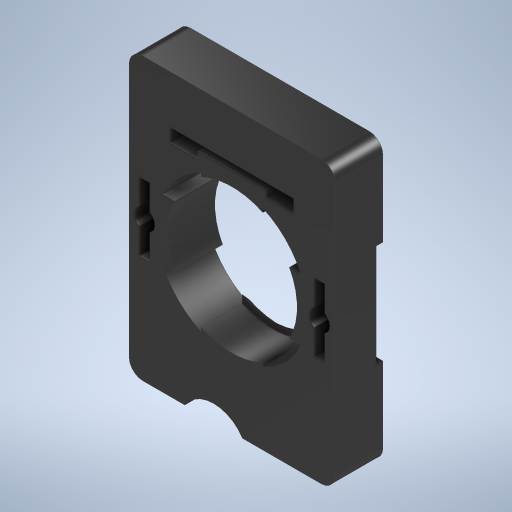
# Autodesk Inventor part: BASE
Saved by Autodesk Inventor 2023 (Build 270158000, 158)
## iProperties
Created: 2023-10-18
Part Number: BASE
Material: Genérico
Document SubType Name: Modeling
Designer: vinicius.sena
Density: 1 g/cm^3
Appearance: Padrão
Author: vinicius.sena
Autodesk Inventor part; units mm, degrees
ref_plane "YZ Plane" through (0, 0, 0) normal (1, 0, 0) x (0, 1, 0)
ref_plane "XZ Plane" through (0, 0, 0) normal (0, 1, 0) x (-1, 0, 0)
ref_plane "XY Plane" through (0, 0, 0) normal (0, 0, 1) x (1, 0, 0)
sketch "Esboço1" plane through (0, 0, 0) normal (0, 0, 1) x (1, 0, 0)
  line L0 (-15, 20.5) -> (15, 20.5)
  line L1 (15, 20.5) -> (15, -20.5)
  line L2 (15, -20.5) -> (-15, -20.5)
  line L3 (-15, -20.5) -> (-15, 20.5)
  line L4 (-15, 20.5) -> (15, -20.5) construction
  line L5 (15, 20.5) -> (-15, -20.5) construction
  point P0 (0, 0)
  dimension "d0" = 30
  dimension "d1" = 41
  constraints: 12 end point, 2 midpoint, 2 parallel, 1 horizontal, 1 perpendicular
  measures "d0" distance of L1.end L2.end
  measures "d1" distance of L0.end L1.end
extrude "Extrusão1" add sketch "Esboço1" along normal blind 7
sketch "Esboço2" plane through (0, 0, 7) normal (0, 0, 1) x (1, 0, 0)
  circle A0 centre (0, 0) radius 11
  dimension "d4" = 22
  constraints: 1 centre point, 1 coincident
  measures "d4" diameter of A0
extrude "Extrusão2" cut sketch "Esboço2" against normal blind 7
sketch "Esboço3" plane through (0, 0, 7) normal (0, 0, 1) x (1, 0, 0)
  circle A0 centre (-2.6743, -23.2026) radius 5
  point P0 (0, 0)
  dimension "d7" = 10
  constraints: 1 centre point
  measures "d7" diameter of A0
extrude "Extrusão3" cut sketch "Esboço3" against normal through all
sketch "Esboço5" plane through (0, 0, 7) normal (0, 0, 1) x (1, 0, 0)
  line L0 (-13.5, 5) -> (-12, 5)
  line L1 (-12, 5) -> (-12, -5)
  line L2 (-12, -5) -> (-13.5, -5)
  line L3 (-13.5, -5) -> (-13.5, 5)
  line L4 (-13.5, 5) -> (-12, -5) construction
  line L5 (-12, 5) -> (-13.5, -5) construction
  line L6 (12, 5) -> (13.5, 5)
  line L7 (13.5, 5) -> (13.5, -5)
  line L8 (13.5, -5) -> (12, -5)
  line L9 (12, -5) -> (12, 5)
  line L10 (12, 5) -> (13.5, -5) construction
  line L11 (13.5, 5) -> (12, -5) construction
  line L12 (15, -20.5) -> (15, 20.5) projected
  line L13 (-15, 20.5) -> (-15, -20.5) projected
  point P0 (0, 0)
  point P1 (-12.75, 0)
  point P2 (12.75, 0)
  dimension "d10" = 1.5
  dimension "d11" = 10
  dimension "d12" = 1.5
  dimension "d13" = 10
  dimension "d14" = 1.5
  dimension "d15" = 1.5
  constraints: 24 end point, 4 midpoint, 4 parallel, 2 horizontal, 2 perpendicular
  measures "d10" distance of L1.end L2.end
  measures "d11" distance of L0.end L1.end
  measures "d12" distance of L7.end L8.end
  measures "d13" distance of L6.end L7.end
  measures "d14" distance between parallel lines of L12 L7
  measures "d15" distance between parallel lines of L13 L3
extrude "Extrusão4" cut sketch "Esboço5" against normal through all
sketch "Esboço6" plane through (0, 0, 7) normal (0, 0, 1) x (1, 0, 0)
  circle A0 centre (12.75, 0) radius 1.5
  circle A1 centre (-12.75, 0) radius 1.5
  line L0 (-13.5, 5) -> (-12, 5) projected
  line L1 (12, 5) -> (13.5, 5) projected
  point P0 (0, 0)
  point P1 (-12.75, 5)
  point P2 (12.75, 5)
  dimension "d18" = 3
  dimension "d19" = 3
  dimension "d20" = 0
  dimension "d21" = 0
  constraints: 2 centre point, 2 midpoint
  measures "d18" diameter of A0
  measures "d19" diameter of A1
  measures "d20" horizontal distance of point (-12.75, 5) A1.centre
  measures "d21" horizontal distance of point (12.75, 5) A0.centre
extrude "Extrusão5" cut sketch "Esboço6" against normal through all
sketch "Esboço7" plane through (0, 0, 7) normal (0, 0, 1) x (1, 0, 0)
  circle A0 centre (0, 0) radius 9.5
  circle A1 centre (0, 0) radius 11
  line L0 (-15, 4.5) -> (15, 4.5)
  line L1 (15, 4.5) -> (15, -4.5)
  line L2 (15, -4.5) -> (-15, -4.5)
  line L3 (-15, -4.5) -> (-15, 4.5)
  line L4 (-15, 4.5) -> (15, -4.5) construction
  line L5 (15, 4.5) -> (-15, -4.5) construction
  line L6 (-4.5, -15) -> (4.5, -15)
  line L7 (4.5, -15) -> (4.5, 15)
  line L8 (4.5, 15) -> (-4.5, 15)
  line L9 (-4.5, 15) -> (-4.5, -15)
  line L10 (-4.5, -15) -> (4.5, 15) construction
  line L11 (4.5, -15) -> (-4.5, 15) construction
  point P0 (8.3666, -4.5)
  point P1 (10.0374, -4.5)
  point P2 (10.0374, 4.5)
  point P3 (8.3666, 4.5)
  point P4 (-4.5, -8.3666)
  point P5 (-4.5, -10.0374)
  point P6 (4.5, -10.0374)
  point P7 (4.5, -8.3666)
  point P8 (-10.0374, -4.5)
  point P9 (-8.3666, -4.5)
  point P10 (-8.3666, 4.5)
  point P11 (-10.0374, 4.5)
  point P12 (-4.5, 10.0374)
  point P13 (-4.5, 8.3666)
  point P14 (4.5, 8.3666)
  point P15 (4.5, 10.0374)
  dimension "d24" = 19
  dimension "d25" = 22
  dimension "d26" = 30
  dimension "d27" = 9
  dimension "d28" = 9
  dimension "d29" = 30
  constraints: 24 end point, 4 midpoint, 4 parallel, 2 centre point, 2 coincident, 2 horizontal, 2 perpendicular
  measures "d24" diameter of A0
  measures "d25" diameter of A1
  measures "d26" distance of L1.end L2.end
  measures "d27" distance of L0.end L1.end
  measures "d28" distance of L8.end L7.end
  measures "d29" distance of L7.end L6.end
extrude "Extrusão6" add sketch "Esboço7" against normal blind 7 contours A0 L0 A1 L2 | A0 L9 A1 L7 | L7 A1 L9 A0 | A0 L2 A1 L0
sketch "Esboço8" plane through (0, 0, 7) normal (0, 0, 1) x (1, 0, 0)
  circle A0 centre (0, 0) radius 11
  circle A1 centre (0, 0) radius 10.5
  circle A2 centre (0, 0) radius 9.5
  line L0 (-4.5, 15) -> (4.5, 15)
  line L1 (4.5, 15) -> (4.5, -15)
  line L2 (4.5, -15) -> (-4.5, -15)
  line L3 (-4.5, -15) -> (-4.5, 15)
  line L4 (-4.5, 15) -> (4.5, -15) construction
  line L5 (4.5, 15) -> (-4.5, -15) construction
  line L6 (-15, 4.5) -> (15, 4.5)
  line L7 (15, 4.5) -> (15, -4.5)
  line L8 (15, -4.5) -> (-15, -4.5)
  line L9 (-15, -4.5) -> (-15, 4.5)
  line L10 (-15, 4.5) -> (15, -4.5) construction
  line L11 (15, 4.5) -> (-15, -4.5) construction
  point P0 (-4.5, -8.3666)
  point P1 (-4.5, -9.4868)
  point P2 (4.5, -9.4868)
  point P3 (4.5, -8.3666)
  point P4 (8.3666, -4.5)
  point P5 (9.4868, -4.5)
  point P6 (9.4868, 4.5)
  point P7 (8.3666, 4.5)
  point P8 (-9.4868, -4.5)
  point P9 (-8.3666, -4.5)
  point P10 (-8.3666, 4.5)
  point P11 (-9.4868, 4.5)
  point P12 (-4.5, 9.4868)
  point P13 (-4.5, 8.3666)
  point P14 (4.5, 8.3666)
  point P15 (4.5, 9.4868)
  dimension "d32" = 22
  dimension "d33" = 21
  dimension "d34" = 19
  dimension "d35" = 9
  dimension "d36" = 30
  dimension "d37" = 30
  dimension "d38" = 9
  constraints: 24 end point, 4 midpoint, 4 parallel, 3 centre point, 3 coincident, 2 horizontal, 2 perpendicular
  measures "d32" diameter of A0
  measures "d33" diameter of A1
  measures "d34" diameter of A2
  measures "d35" distance of L1.end L2.end
  measures "d36" distance of L0.end L1.end
  measures "d37" distance of L7.end L8.end
  measures "d38" distance of L6.end L7.end
extrude "Extrusão7" cut sketch "Esboço8" against normal blind 6 contours L1 A2 L3 A1 | A1 L3 A2 L1
chamfer "Chanfro1" distance 1 angle 45 2 edges at (0, -9.5, 0) (0, 9.5, 0)
sketch "Esboço9" plane through (0, 0, 0) normal (0, 0, -1) x (-1, 0, 0)
  line L0 (15.25, 7.5) -> (10.25, 7.5)
  line L1 (10.25, 7.5) -> (10.25, -7.5)
  line L2 (10.25, -7.5) -> (15.25, -7.5)
  line L3 (15.25, -7.5) -> (15.25, 7.5)
  arc A0 (13.5, -1.299) -> (13.5, 1.299) centre (12.75, 0) ccw projected
  line L4 (15.25, 7.5) -> (10.25, -7.5) construction
  line L5 (10.25, 7.5) -> (15.25, -7.5) construction
  line L6 (-10.25, 7.5) -> (-15.25, 7.5)
  line L7 (-15.25, 7.5) -> (-15.25, -7.5)
  line L8 (-15.25, -7.5) -> (-10.25, -7.5)
  line L9 (-10.25, -7.5) -> (-10.25, 7.5)
  arc A1 (-12, -1.299) -> (-12, 1.299) centre (-12.75, 0) ccw projected
  line L10 (-10.25, 7.5) -> (-15.25, -7.5) construction
  line L11 (-15.25, 7.5) -> (-10.25, -7.5) construction
  point P0 (0, 0)
  dimension "d44" = 5
  dimension "d45" = 15
  dimension "d46" = 5
  dimension "d47" = 15
  constraints: 24 end point, 4 midpoint, 4 parallel, 2 horizontal, 2 perpendicular
  measures "d44" distance of L2.end L1.end
  measures "d45" distance of L1.end L0.end
  measures "d46" distance of L8.end L7.end
  measures "d47" distance of L7.end L6.end
extrude "Extrusão8" cut sketch "Esboço9" against normal blind 1
fillet "Arredondamento1" radius 2 4 edges at (-15, -20.5, 3.5) (15, -20.5, 3.5) (15, 20.5, 3.5) (-15, 20.5, 3.5)
sketch "Esboço10" plane through (0, 0, 7) normal (0, 0, 1) x (1, 0, 0)
  line L0 (-9, 13.5) -> (9, 13.5)
  line L1 (9, 13.5) -> (9, 12.5)
  line L2 (9, 12.5) -> (-9, 12.5)
  line L3 (-9, 12.5) -> (-9, 13.5)
  line L4 (-9, 13.5) -> (9, 12.5) construction
  line L5 (9, 13.5) -> (-9, 12.5) construction
  arc A0 (4.5, 9.4868) -> (-4.5, 9.4868) centre (0, 0) ccw projected
  point P0 (0, 13)
  point P1 (0, 10.5)
  point P2 (0, 12.5)
  dimension "d51" = 18
  dimension "d52" = 1
  dimension "d53" = 2
  constraints: 12 end point, 3 midpoint, 2 parallel, 1 horizontal, 1 perpendicular, 1 point on circle
  measures "d51" distance of L1.end L2.end
  measures "d52" distance of L0.end L1.end
  measures "d53" distance of point (0, 10.5) point (0, 12.5)
extrude "Extrusão9" cut sketch "Esboço10" against normal through all
sketch "Esboço11" plane through (0, 0, 7) normal (0, 0, 1) x (1, 0, 0)
  line L0 (5, 12.5) -> (9, 12.5)
  line L1 (9, 12.5) -> (9, 11.5)
  line L2 (9, 11.5) -> (5, 11.5)
  line L3 (5, 11.5) -> (5, 12.5)
  line L4 (5, 12.5) -> (9, 11.5) construction
  line L5 (9, 12.5) -> (5, 11.5) construction
  line L6 (-9, 12.5) -> (-5, 12.5)
  line L7 (-5, 12.5) -> (-5, 11.5)
  line L8 (-5, 11.5) -> (-9, 11.5)
  line L9 (-9, 11.5) -> (-9, 12.5)
  line L10 (-9, 12.5) -> (-5, 11.5) construction
  line L11 (-5, 12.5) -> (-9, 11.5) construction
  line L12 (9, 12.5) -> (-9, 12.5) projected
  line L13 (-9, 12.5) -> (-9, 13.5) projected
  line L14 (9, 13.5) -> (9, 12.5) projected
  point P0 (0, 0)
  point P1 (7, 12)
  point P2 (-7, 12)
  point P3 (-9, 13)
  point P4 (-9, 12)
  point P5 (9, 13)
  point P6 (9, 12)
  dimension "d56" = 4
  dimension "d57" = 1
  dimension "d58" = 4
  dimension "d59" = 1
  dimension "d60" = 0
  dimension "d61" = 0
  dimension "d62" = 0
  dimension "d63" = 0
  constraints: 24 end point, 8 midpoint, 4 parallel, 2 horizontal, 2 perpendicular
  measures "d56" distance of L1.end L2.end
  measures "d57" distance of L0.end L1.end
  measures "d58" distance of L7.end L8.end
  measures "d59" distance of L6.end L7.end
  measures "d60" distance between parallel lines of L12 L6
  measures "d61" horizontal distance of point (-9, 13) point (-9, 12)
  measures "d62" distance between parallel lines of L12 L0
  measures "d63" horizontal distance of point (9, 13) point (9, 12)
extrude "Extrusão10" cut sketch "Esboço11" against normal blind 10
sketch "Esboço12" plane through (0, 0, 0) normal (0, 0, -1) x (-1, 0, 0)
  line L0 (3, -17.642) -> (-3, -17.642)
  line L1 (-3, -17.642) -> (-3, -12.642)
  line L2 (-3, -12.642) -> (3, -12.642)
  line L3 (3, -12.642) -> (3, -17.642)
  line L4 (3, -17.642) -> (-3, -12.642) construction
  line L5 (-3, -17.642) -> (3, -12.642) construction
  line L6 (-7, -18.642) -> (-14, -18.642)
  line L7 (-14, -18.642) -> (-14, -11.642)
  line L8 (-14, -11.642) -> (-7, -11.642)
  line L9 (-7, -11.642) -> (-7, -18.642)
  line L10 (-7, -18.642) -> (-14, -11.642) construction
  line L11 (-14, -18.642) -> (-7, -11.642) construction
  line L12 (14, -18.642) -> (7, -18.642)
  line L13 (7, -18.642) -> (7, -11.642)
  line L14 (7, -11.642) -> (14, -11.642)
  line L15 (14, -11.642) -> (14, -18.642)
  line L16 (14, -18.642) -> (7, -11.642) construction
  line L17 (7, -18.642) -> (14, -11.642) construction
  line L18 (6, -18.142) -> (4, -18.142)
  line L19 (4, -18.142) -> (4, -12.142)
  line L20 (4, -12.142) -> (6, -12.142)
  line L21 (6, -12.142) -> (6, -18.142)
  line L22 (6, -18.142) -> (4, -12.142) construction
  line L23 (4, -18.142) -> (6, -12.142) construction
  line L24 (-4, -18.142) -> (-6, -18.142)
  line L25 (-6, -18.142) -> (-6, -12.142)
  line L26 (-6, -12.142) -> (-4, -12.142)
  line L27 (-4, -12.142) -> (-4, -18.142)
  line L28 (-4, -18.142) -> (-6, -12.142) construction
  line L29 (-6, -18.142) -> (-4, -12.142) construction
  line L30 (15, -7.5) -> (15, -18.5) projected
  line L31 (-15, -18.5) -> (-15, -7.5) projected
  point P0 (0, 0)
  point P1 (0, -15.142)
  point P2 (-10.5, -15.142)
  point P3 (10.5, -15.142)
  point P4 (5, -15.142)
  point P5 (-5, -15.142)
  point P6 (14, -15.142)
  dimension "d66" = 6
  dimension "d67" = 5
  dimension "d68" = 7
  dimension "d69" = 7
  dimension "d70" = 7
  dimension "d71" = 7
  dimension "d72" = 2
  dimension "d73" = 6
  dimension "d74" = 2
  dimension "d75" = 6
  dimension "d76" = 1
  dimension "d77" = 1
  dimension "d78" = 5.5
  dimension "d79" = 5.5
  constraints: 60 end point, 11 midpoint, 10 parallel, 5 horizontal, 5 perpendicular
  measures "d66" distance of L1.end L2.end
  measures "d67" distance of L0.end L1.end
  measures "d68" distance of L7.end L8.end
  measures "d69" distance of L6.end L7.end
  measures "d70" distance of L13.end L14.end
  measures "d71" distance of L12.end L13.end
  measures "d72" distance of L19.end L20.end
  measures "d73" distance of L18.end L19.end
  measures "d74" distance of L25.end L26.end
  measures "d75" distance of L24.end L25.end
  measures "d76" distance from line of L30 point (14, -15.142)
  measures "d77" distance between parallel lines of L31 L7
  measures "d78" distance of point (-5, -15.142) point (-10.5, -15.142)
  measures "d79" distance of point (10.5, -15.142) point (5, -15.142)
extrude "Extrusão11" cut sketch "Esboço12" against normal blind 6
sketch "Esboço13" plane through (0, 0, 0) normal (0, 0, -1) x (-1, 0, 0)
  line L0 (3.5, 14.5253) -> (-3.5, 14.5253)
  line L1 (-3.5, 14.5253) -> (-3.5, 19.5253)
  line L2 (-3.5, 19.5253) -> (3.5, 19.5253)
  line L3 (3.5, 19.5253) -> (3.5, 14.5253)
  line L4 (3.5, 14.5253) -> (-3.5, 19.5253) construction
  line L5 (-3.5, 14.5253) -> (3.5, 19.5253) construction
  line L6 (-5, 14.5253) -> (-10, 14.5253)
  line L7 (-10, 14.5253) -> (-10, 19.5253)
  line L8 (-10, 19.5253) -> (-5, 19.5253)
  line L9 (-5, 19.5253) -> (-5, 14.5253)
  line L10 (-5, 14.5253) -> (-10, 19.5253) construction
  line L11 (-10, 14.5253) -> (-5, 19.5253) construction
  line L12 (10, 14.5253) -> (5, 14.5253)
  line L13 (5, 14.5253) -> (5, 19.5253)
  line L14 (5, 19.5253) -> (10, 19.5253)
  line L15 (10, 19.5253) -> (10, 14.5253)
  line L16 (10, 14.5253) -> (5, 19.5253) construction
  line L17 (5, 14.5253) -> (10, 19.5253) construction
  line L18 (13.5, 8.4846) -> (11.5, 8.4846)
  line L19 (11.5, 8.4846) -> (11.5, 18.4846)
  line L20 (11.5, 18.4846) -> (13.5, 18.4846)
  line L21 (13.5, 18.4846) -> (13.5, 8.4846)
  line L22 (13.5, 8.4846) -> (11.5, 18.4846) construction
  line L23 (11.5, 8.4846) -> (13.5, 18.4846) construction
  line L24 (-11.5, 8.6427) -> (-13.5, 8.6427)
  line L25 (-13.5, 8.6427) -> (-13.5, 18.6427)
  line L26 (-13.5, 18.6427) -> (-11.5, 18.6427)
  line L27 (-11.5, 18.6427) -> (-11.5, 8.6427)
  line L28 (-11.5, 8.6427) -> (-13.5, 18.6427) construction
  line L29 (-13.5, 8.6427) -> (-11.5, 18.6427) construction
  point P0 (0, 0)
  point P1 (0, 17.0253)
  point P2 (-7.5, 17.0253)
  point P3 (7.5, 17.0253)
  point P4 (12.5, 13.4846)
  point P5 (-12.5, 13.6427)
  dimension "d82" = 7
  dimension "d83" = 5
  dimension "d84" = 5
  dimension "d85" = 5
  dimension "d86" = 5
  dimension "d87" = 5
  dimension "d88" = 2
  dimension "d89" = 10
  dimension "d90" = 2
  dimension "d91" = 10
  dimension "d92" = 7.5
  dimension "d93" = 7.5
  dimension "d94" = 5
  dimension "d95" = 5
  constraints: 60 end point, 10 midpoint, 10 parallel, 5 horizontal, 5 perpendicular
  measures "d82" distance of L1.end L2.end
  measures "d83" distance of L0.end L1.end
  measures "d84" distance of L7.end L8.end
  measures "d85" distance of L6.end L7.end
  measures "d86" distance of L13.end L14.end
  measures "d87" distance of L12.end L13.end
  measures "d88" distance of L19.end L20.end
  measures "d89" distance of L18.end L19.end
  measures "d90" distance of L25.end L26.end
  measures "d91" distance of L24.end L25.end
  measures "d92" distance of point (0, 17.025) point (-7.5, 17.025)
  measures "d93" distance of point (0, 17.025) point (7.5, 17.025)
  measures "d94" horizontal distance of point (7.5, 17.025) point (12.5, 13.485)
  measures "d95" horizontal distance of point (-7.5, 17.025) point (-12.5, 13.643)
extrude "Extrusão12" cut sketch "Esboço13" against normal blind 6
fillet "Arredondamento2" radius 1 20 edges at (14, -18.642, 3) (7, -18.642, 3) (4, -18.142, 3) (6, -18.142, 3) (6, -12.142, 3) (4, -12.142, 3) (7, -11.642, 3) (14, -11.642, 3) (3, -12.642, 3) (3, -17.642, 3) (-3, -17.642, 3) (-3, -12.642, 3) (-6, -12.142, 3) (-4, -12.142, 3) (-6, -18.142, 3) (-4, -18.142, 3) (-7, -18.642, 3) (-14, -18.642, 3) (-14, -11.642, 3) (-7, -11.642, 3)
fillet "Arredondamento3" radius 1 20 edges at (11.5, 8.6427, 3) (13.5, 8.6427, 3) (11.5, 18.6427, 3) (13.5, 18.6427, 3) (5, 14.5253, 3) (10, 14.5253, 3) (5, 19.5253, 3) (10, 19.5253, 3) (3.5, 14.5253, 3) (-3.5, 14.5253, 3) (-3.5, 19.5253, 3) (3.5, 19.5253, 3) (-5, 19.5253, 3) (-5, 14.5253, 3) (-10, 14.5253, 3) (-10, 19.5253, 3) (-13.5, 18.4846, 3) (-11.5, 18.4846, 3) (-11.5, 8.4846, 3) (-13.5, 8.4846, 3)
